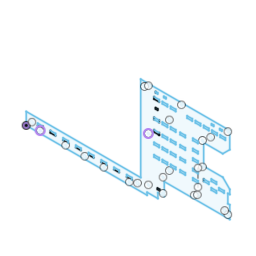
R&S UPL KeyBoard BackPanel (Autodesk Fusion 360 design; units mm, degrees)
description: Rohde & Schwarz UPL
Autodesk Fusion 360 part; units mm, degrees
sketch "Mechanical Outline" plane through (0, 0, 0) normal (0, 0, 1) x (1, 0, 0)
  line L0 (180, 19) -> (0, 19)
  line L1 (309, 116) -> (279, 116)
  line L2 (279, 116) -> (279, 84)
  line L3 (279, 84) -> (309, 84)
  line L4 (309, 84) -> (320, 73)
  line L5 (320, 66) -> (317, 66)
  line L6 (317, 66) -> (317, 52)
  line L7 (317, 52) -> (320, 52)
  line L8 (320, 66) -> (320, 73)
  line L9 (320, 32) -> (217, 32)
  line L10 (190, 0) -> (0, 0)
  line L11 (0, 19) -> (0, 0)
  line L12 (320, 52) -> (320, 32)
  line L13 (207, 4) -> (190, 4)
  line L14 (190, 4) -> (190, 0)
  line L15 (207, 12) -> (217, 12)
  line L16 (207, 12) -> (207, 4)
  line L17 (217, 32) -> (217, 12)
  line L18 (320, 153) -> (180, 153)
  line L19 (180, 19) -> (180, 153)
  line L20 (320, 153) -> (320, 127)
  line L21 (309, 116) -> (320, 127)
  dimension "d21" = 3
  dimension "d22" = 14
  dimension "d124" = 19
  dimension "d126" = 103
  dimension "d130" = 4
  dimension "d131" = 8
  dimension "d132" = 20
  dimension "d133" = 17
  dimension "d134" = 10
  constraint horizontal L1
  constraint vertical L2
  constraint horizontal L3
  constraint horizontal L5
  constraint vertical L6
  constraint horizontal L7
  constraint horizontal L9
  constraint horizontal L10
  constraint perpendicular L10 L11
  constraint horizontal L13
  constraint perpendicular L10 L14
  constraint horizontal L15
  constraint horizontal L18
  constraint perpendicular L18 L19
  measures "d21" distance of L5.start L5.end
  measures "d22" distance of L5.start L7.end
  measures "d124" distance of L0.end L10.end
  measures "d126" distance of L9.start L9.end
  measures "d130" distance of L10.start L13.end
  measures "d131" distance of L13.start L15.start
  measures "d132" distance of L9.end L15.end
  measures "d133" distance of L13.start L13.end
  measures "d134" distance of L15.start L15.end
sketch "Holes" plane through (0, 0, 0) normal (0, 0, 1) x (1, 0, 0)
  circle A0 centre (175, 9) radius 2
  circle A1 centre (186, 146) radius 2
  circle A2 centre (92, 4) radius 2
  circle A3 centre (9, 9) radius 2
  circle A4 centre (22, 4) radius 1.25
  circle A5 centre (62, 4) radius 1.25
  circle A6 centre (122, 4) radius 1.25
  circle A7 centre (162, 4) radius 1.25
  circle A8 centre (192, 150) radius 1.25
  circle A9 centre (192, 85) radius 1.25
  circle A10 centre (192, 15) radius 1.25
  circle A11 centre (244, 150) radius 1.25
  circle A12 centre (317, 150) radius 1.25
  circle A13 centre (225, 120) radius 2
  circle A14 centre (290, 129) radius 2
  circle A15 centre (225, 51) radius 2
  circle A16 centre (277, 118) radius 1.25
  circle A17 centre (277, 82) radius 1.25
  circle A18 centre (215, 15) radius 1.25
  circle A19 centre (215, 37) radius 1.25
  circle A20 centre (264, 37) radius 1.25
  circle A21 centre (317, 37) radius 1.25
  circle A22 centre (269, 40) radius 2
  circle A23 centre (312, 40) radius 2
  dimension "d28" = 4
  dimension "d31" = 4
  dimension "d39" = 4
  dimension "d40" = 4
  dimension "d41" = 2.5
  dimension "d43" = 2.5
  dimension "d44" = 2.5
  dimension "d51" = 13
  dimension "d52" = 40
  dimension "d53" = 30
  dimension "d55" = 40
  dimension "d56" = 13
  dimension "d60" = 2.5
  dimension "d61" = 6
  dimension "d62" = 4
  dimension "d63" = 2.5
  dimension "d66" = 2.5
  dimension "d69" = 2.5
  dimension "d70" = 2.5
  dimension "d73" = 52
  dimension "d75" = 4
  dimension "d76" = 4
  dimension "d77" = 4
  dimension "d78" = 39
  dimension "d79" = 104
  dimension "d80" = 17
  dimension "d81" = 26
  dimension "d82" = 95
  dimension "d84" = 2.5
  dimension "d85" = 2.5
  dimension "d86" = 91
  dimension "d88" = 28
  dimension "d89" = 64
  dimension "d90" = 2.5
  dimension "d91" = 2.5
  dimension "d92" = 2.5
  dimension "d93" = 2.5
  dimension "d94" = 4
  dimension "d95" = 4
  dimension "d111" = 60
  dimension "d112" = 65
  dimension "d113" = 70
  dimension "d114" = 73
  dimension "d115" = 22
  dimension "d116" = 49
  dimension "d117" = 53
  dimension "d118" = 23
  dimension "d119" = 44
  dimension "d120" = 43
  dimension "d121" = 11
  dimension "d122" = 2.5
  constraint horizontal A10.centre A18.centre
  constraint vertical A18.centre A19.centre
  constraint horizontal A19.centre A20.centre
  constraint horizontal A20.centre A21.centre
  constraint vertical A16.centre A17.centre
  constraint horizontal A6.centre A7.centre
  constraint horizontal A4.centre A5.centre
  constraint horizontal A0.centre A3.centre
  constraint horizontal A8.centre A11.centre
  constraint horizontal A11.centre A12.centre
  constraint vertical A13.centre A15.centre
  constraint vertical A8.centre A9.centre
  constraint horizontal A22.centre A23.centre
  measures "d28" diameter of A0
  measures "d31" diameter of A1
  measures "d39" diameter of A2
  measures "d40" diameter of A3
  measures "d41" diameter of A4
  measures "d43" diameter of A6
  measures "d44" diameter of A7
  measures "d51" horizontal distance of A0.centre A7.centre
  measures "d52" distance of A6.centre A7.centre
  measures "d53" horizontal distance of A2.centre A6.centre
  measures "d55" distance of A4.centre A5.centre
  measures "d56" horizontal distance of A3.centre A4.centre
  measures "d60" diameter of A8
  measures "d61" horizontal distance of A1.centre A8.centre
  measures "d62" vertical distance of A1.centre A8.centre
  measures "d63" diameter of A9
  measures "d66" diameter of A10
  measures "d69" diameter of A11
  measures "d70" diameter of A12
  measures "d73" distance of A8.centre A11.centre
  measures "d75" diameter of A13
  measures "d76" diameter of A14
  measures "d77" diameter of A15
  measures "d78" horizontal distance of A1.centre A13.centre
  measures "d79" horizontal distance of A1.centre A14.centre
  measures "d80" vertical distance of A1.centre A14.centre
  measures "d81" vertical distance of A1.centre A13.centre
  measures "d82" vertical distance of A1.centre A15.centre
  measures "d84" diameter of A16
  measures "d85" diameter of A17
  measures "d86" horizontal distance of A1.centre A16.centre
  measures "d88" vertical distance of A1.centre A16.centre
  measures "d89" vertical distance of A1.centre A17.centre
  measures "d90" diameter of A18
  measures "d91" diameter of A19
  measures "d92" diameter of A20
  measures "d93" diameter of A21
  measures "d94" diameter of A22
  measures "d95" diameter of A23
  measures "d111" distance of A5.centre A6.centre
  measures "d112" distance of A8.centre A9.centre
  measures "d113" distance of A9.centre A10.centre
  measures "d114" distance of A11.centre A12.centre
  measures "d115" distance of A18.centre A19.centre
  measures "d116" distance of A19.centre A20.centre
  measures "d117" distance of A20.centre A21.centre
  measures "d118" distance of A10.centre A18.centre
  measures "d119" horizontal distance of A15.centre A22.centre
  measures "d120" distance of A22.centre A23.centre
  measures "d121" vertical distance of A15.centre A22.centre
  measures "d122" diameter of A5
extrude "Extrude1" add sketch "Mechanical Outline" along normal blind 1
sketch "Buttons/Leds" plane through (0, 0, 0) normal (0, 0, 1) x (1, 0, 0)
  line L0 (26, 12) -> (26, 9)
  line L1 (58, 9) -> (66, 9)
  line L2 (106, 12) -> (106, 9)
  line L3 (86, 12) -> (86, 9)
  line L4 (66, 12) -> (58, 12)
  line L5 (46, 9) -> (38, 9)
  line L6 (26, 9) -> (18, 9)
  line L7 (86, 9) -> (78, 9)
  line L8 (66, 9) -> (66, 12)
  line L9 (18, 9) -> (18, 12)
  line L10 (106, 9) -> (98, 9)
  line L11 (138, 12) -> (146, 12)
  line L12 (146, 12) -> (146, 9)
  line L13 (118, 12) -> (126, 12)
  line L14 (138, 9) -> (138, 12)
  line L15 (158, 9) -> (158, 12)
  line L16 (166, 12) -> (166, 9)
  line L17 (98, 12) -> (106, 12)
  line L18 (126, 12) -> (126, 9)
  line L19 (158, 12) -> (166, 12)
  line L20 (146, 9) -> (138, 9)
  line L21 (166, 9) -> (158, 9)
  line L22 (18, 12) -> (26, 12)
  line L23 (78, 9) -> (78, 12)
  line L24 (78, 12) -> (86, 12)
  line L25 (58, 12) -> (58, 9)
  line L26 (38, 9) -> (38, 12)
  line L27 (46, 12) -> (46, 9)
  line L28 (38, 12) -> (46, 12)
  line L29 (98, 9) -> (98, 12)
  line L30 (126, 9) -> (118, 9)
  line L31 (118, 9) -> (118, 12)
  line L32 (214, 111.5) -> (222, 111.5)
  line L33 (227, 77.5) -> (235, 77.5)
  line L34 (242, 108.5) -> (242, 111.5)
  line L35 (235, 108.5) -> (227, 108.5)
  line L36 (235, 74.5) -> (227, 74.5)
  line L37 (250, 94.5) -> (250, 91.5)
  line L38 (235, 91.5) -> (227, 91.5)
  line L39 (222, 60.5) -> (222, 57.5)
  line L40 (270, 110.5) -> (262, 110.5)
  line L41 (270, 96.5) -> (262, 96.5)
  line L42 (262, 83.5) -> (262, 86.5)
  line L43 (262, 113.5) -> (270, 113.5)
  line L44 (262, 96.5) -> (262, 99.5)
  line L45 (262, 110.5) -> (262, 113.5)
  line L46 (270, 59.5) -> (270, 56.5)
  line L47 (270, 99.5) -> (270, 96.5)
  line L48 (262, 69.5) -> (262, 72.5)
  line L49 (270, 72.5) -> (270, 69.5)
  line L50 (262, 59.5) -> (270, 59.5)
  line L51 (262, 86.5) -> (270, 86.5)
  line L52 (270, 69.5) -> (262, 69.5)
  line L53 (270, 86.5) -> (270, 83.5)
  line L54 (262, 72.5) -> (270, 72.5)
  line L55 (270, 56.5) -> (262, 56.5)
  line L56 (270, 83.5) -> (262, 83.5)
  line L57 (262, 56.5) -> (262, 59.5)
  line L58 (270, 113.5) -> (270, 110.5)
  line L59 (262, 99.5) -> (270, 99.5)
  line L60 (250, 57.5) -> (242, 57.5)
  line L61 (242, 111.5) -> (250, 111.5)
  line L62 (209, 77.5) -> (209, 74.5)
  line L63 (242, 60.5) -> (250, 60.5)
  line L64 (227, 111.5) -> (235, 111.5)
  line L65 (201, 94.5) -> (209, 94.5)
  line L66 (227, 60.5) -> (235, 60.5)
  line L67 (201, 77.5) -> (209, 77.5)
  line L68 (235, 57.5) -> (227, 57.5)
  line L69 (214, 74.5) -> (214, 77.5)
  line L70 (222, 108.5) -> (214, 108.5)
  line L71 (222, 111.5) -> (222, 108.5)
  line L72 (214, 60.5) -> (222, 60.5)
  line L73 (222, 91.5) -> (214, 91.5)
  line L74 (250, 111.5) -> (250, 108.5)
  line L75 (227, 108.5) -> (227, 111.5)
  line L76 (222, 94.5) -> (222, 91.5)
  line L77 (222, 57.5) -> (214, 57.5)
  line L78 (250, 74.5) -> (242, 74.5)
  line L79 (209, 60.5) -> (209, 57.5)
  line L80 (227, 57.5) -> (227, 60.5)
  line L81 (209, 91.5) -> (201, 91.5)
  line L82 (235, 60.5) -> (235, 57.5)
  line L83 (235, 94.5) -> (235, 91.5)
  line L84 (214, 57.5) -> (214, 60.5)
  line L85 (201, 57.5) -> (201, 60.5)
  line L86 (201, 60.5) -> (209, 60.5)
  line L87 (250, 91.5) -> (242, 91.5)
  line L88 (209, 57.5) -> (201, 57.5)
  line L89 (201, 111.5) -> (209, 111.5)
  line L90 (209, 111.5) -> (209, 108.5)
  line L91 (201, 74.5) -> (201, 77.5)
  line L92 (214, 108.5) -> (214, 111.5)
  line L93 (242, 91.5) -> (242, 94.5)
  line L94 (242, 57.5) -> (242, 60.5)
  line L95 (250, 108.5) -> (242, 108.5)
  line L96 (214, 91.5) -> (214, 94.5)
  line L97 (235, 111.5) -> (235, 108.5)
  line L98 (250, 60.5) -> (250, 57.5)
  line L99 (214, 77.5) -> (222, 77.5)
  line L100 (209, 94.5) -> (209, 91.5)
  line L101 (209, 108.5) -> (201, 108.5)
  line L102 (209, 74.5) -> (201, 74.5)
  line L103 (201, 108.5) -> (201, 111.5)
  line L104 (222, 74.5) -> (214, 74.5)
  line L105 (227, 74.5) -> (227, 77.5)
  line L106 (227, 91.5) -> (227, 94.5)
  line L107 (222, 77.5) -> (222, 74.5)
  line L108 (235, 77.5) -> (235, 74.5)
  line L109 (242, 94.5) -> (250, 94.5)
  line L110 (250, 77.5) -> (250, 74.5)
  line L111 (242, 77.5) -> (250, 77.5)
  line L112 (214, 94.5) -> (222, 94.5)
  line L113 (227, 94.5) -> (235, 94.5)
  line L114 (242, 74.5) -> (242, 77.5)
  line L115 (201, 94.5) -> (201, 91.5)
  line L116 (209, 91.5) -> (208.5, 91.5)
  line L117 (291, 69.5) -> (291, 72.5)
  line L118 (311, 63.5) -> (303, 63.5)
  line L119 (270, 77) -> (270, 51) construction
  line L120 (279, 66.5) -> (287, 66.5)
  line L121 (287, 66.5) -> (287, 63.5)
  line L122 (287, 63.5) -> (279, 63.5)
  line L123 (279, 63.5) -> (279, 66.5)
  line L124 (291, 72.5) -> (299, 72.5)
  line L125 (299, 72.5) -> (299, 69.5)
  line L126 (291, 60.5) -> (299, 60.5)
  line L127 (299, 60.5) -> (299, 57.5)
  line L128 (299, 57.5) -> (291, 57.5)
  line L129 (303, 66.5) -> (311, 66.5)
  line L130 (311, 66.5) -> (311, 63.5)
  line L131 (291, 57.5) -> (291, 60.5)
  line L132 (291, 69.5) -> (299, 69.5)
  line L133 (303, 66.5) -> (303, 63.5)
  line L134 (235, 139.5) -> (235, 136.5)
  line L135 (227, 139.5) -> (235, 139.5)
  line L136 (235, 136.5) -> (227, 136.5)
  line L137 (274, 139.5) -> (274, 136.5)
  line L138 (222, 136.5) -> (222, 139.5)
  line L139 (227, 136.5) -> (227, 139.5)
  line L140 (201, 136.5) -> (201, 139.5)
  line L141 (203.4, 146.2) -> (203.4, 147.8)
  line L142 (214, 139.5) -> (214, 136.5)
  line L143 (266, 136.5) -> (266, 139.5)
  line L144 (304.4, 146.2) -> (304.4, 147.8)
  line L145 (294.6, 147.8) -> (294.6, 146.2)
  line L146 (253, 136.5) -> (253, 139.5)
  line L147 (287, 139.5) -> (287, 136.5)
  line L148 (206.6, 147.8) -> (206.6, 146.2)
  line L149 (266, 139.5) -> (274, 139.5)
  line L150 (279, 139.5) -> (287, 139.5)
  line L151 (209, 136.5) -> (201, 136.5)
  line L152 (216.4, 146.2) -> (216.4, 147.8)
  line L153 (219.6, 147.8) -> (219.6, 146.2)
  line L154 (216.4, 147.8) -> (219.6, 147.8)
  line L155 (307.6, 146.2) -> (304.4, 146.2)
  line L156 (201, 139.5) -> (209, 139.5)
  line L157 (305, 139.5) -> (313, 139.5)
  line L158 (219.6, 146.2) -> (216.4, 146.2)
  line L159 (203.4, 147.8) -> (206.6, 147.8)
  line L160 (206.6, 146.2) -> (203.4, 146.2)
  line L161 (209, 139.5) -> (209, 136.5)
  line L162 (287, 136.5) -> (279, 136.5)
  line L163 (291.4, 147.8) -> (294.6, 147.8)
  line L164 (292, 136.5) -> (292, 139.5)
  line L165 (274, 136.5) -> (266, 136.5)
  line L166 (253, 139.5) -> (261, 139.5)
  line L167 (300, 136.5) -> (292, 136.5)
  line L168 (294.6, 146.2) -> (291.4, 146.2)
  line L169 (291.4, 146.2) -> (291.4, 147.8)
  line L170 (261, 136.5) -> (253, 136.5)
  line L171 (279, 136.5) -> (279, 139.5)
  line L172 (313, 139.5) -> (313, 136.5)
  line L173 (307.6, 147.8) -> (307.6, 146.2)
  line L174 (222, 139.5) -> (214, 139.5)
  line L175 (313, 136.5) -> (305, 136.5)
  line L176 (214, 136.5) -> (222, 136.5)
  line L177 (261, 139.5) -> (261, 136.5)
  line L178 (305, 136.5) -> (305, 139.5)
  line L179 (292, 139.5) -> (300, 139.5)
  line L180 (300, 139.5) -> (300, 136.5)
  line L181 (304.4, 147.8) -> (307.6, 147.8)
  line L182 (206.6, 125.8) -> (203.4, 125.8)
  line L183 (203.4, 125.8) -> (203.4, 124.2)
  line L184 (203.4, 124.2) -> (206.6, 124.2)
  line L185 (206.6, 124.2) -> (206.6, 125.8)
  line L186 (209.6, 16.2) -> (209.6, 17.8)
  line L187 (206.4, 17.8) -> (206.4, 16.2)
  line L188 (209.6, 17.8) -> (206.4, 17.8)
  line L189 (206.4, 16.2) -> (209.6, 16.2)
  point P0 (22, 4)
  point P1 (192, 85)
  dimension "d142" = 4
  dimension "d143" = 5
  dimension "d144" = 5
  dimension "d145" = 12
  dimension "d147" = 12
  dimension "d148" = 5
  dimension "d149" = 12
  dimension "d150" = 5
  dimension "d151" = 12
  dimension "d153" = 5
  dimension "d154" = 12
  dimension "d155" = 5
  dimension "d156" = 12
  dimension "d157" = 5
  dimension "d158" = 12
  dimension "d159" = 5
  dimension "d160" = 5
  dimension "d161" = 5
  dimension "d162" = 5
  dimension "d163" = 5
  dimension "d164" = 5
  dimension "d165" = 5
  dimension "d166" = 5
  dimension "d167" = 5
  dimension "d168" = 7
  dimension "d169" = 7
  dimension "d170" = 7
  dimension "d171" = 7
  dimension "d172" = 12
  dimension "d173" = 12
  dimension "d174" = 12
  dimension "d175" = 12
  dimension "d176" = 12
  dimension "d177" = 14
  dimension "d178" = 14
  dimension "d179" = 14
  dimension "d180" = 14
  dimension "d181" = 14
  dimension "d182" = 14
  dimension "d183" = 14
  dimension "d184" = 14
  dimension "d185" = 14
  dimension "d186" = 14
  dimension "d187" = 14
  dimension "d188" = 14
  dimension "d189" = 11
  dimension "d190" = 10
  dimension "d191" = 11
  dimension "d192" = 10
  dimension "d193" = 2
  dimension "d194" = 5
  dimension "d195" = 9
  dimension "d196" = 12
  dimension "d197" = 1
  dimension "d198" = 6.5
  dimension "d199" = 9
  dimension "d244" = 8
  dimension "d245" = 3
  dimension "d248" = 8
  dimension "d249" = 8
  dimension "d250" = 8
  dimension "d251" = 8
  dimension "d252" = 8
  dimension "d253" = 8
  dimension "d254" = 8
  dimension "d255" = 8
  dimension "d256" = 8
  dimension "d257" = 8
  dimension "d258" = 8
  dimension "d259" = 8
  dimension "d260" = 8
  dimension "d261" = 8
  dimension "d262" = 8
  dimension "d263" = 8
  dimension "d264" = 8
  dimension "d265" = 8
  dimension "d266" = 8
  dimension "d267" = 8
  dimension "d268" = 3
  dimension "d269" = 3
  dimension "d270" = 3
  dimension "d271" = 3
  dimension "d274" = 3
  dimension "d275" = 3
  dimension "d276" = 9
  dimension "d278" = 12
  dimension "d279" = 78
  dimension "d281" = 9
  dimension "d282" = 4
  dimension "d283" = 4
  dimension "d284" = 4
  dimension "d285" = 4
  dimension "d286" = 3
  dimension "d287" = 3
  dimension "d288" = 3
  dimension "d289" = 3
  dimension "d290" = 3
  dimension "d291" = 6.7
  dimension "d292" = 6.7
  dimension "d293" = 6.7
  dimension "d294" = 6.7
  dimension "d295" = 2.4
  dimension "d296" = 5
  dimension "d297" = 5
  dimension "d298" = 9.8
  dimension "d299" = 18
  dimension "d300" = 5
  dimension "d301" = 5
  dimension "d302" = 5
  dimension "d303" = 5
  dimension "d305" = 9
  dimension "d306" = 51.5
  dimension "d307" = 3.2
  dimension "d308" = 1.6
  dimension "d309" = 10.7
  dimension "d311" = 2.4
  dimension "d312" = 3.2
  dimension "d313" = 1.6
  dimension "d314" = 67.2
  dimension "d315" = 14.4
  dimension "d317" = 71.8
  dimension "d318" = 9.8
  constraint horizontal L6
  constraint horizontal L5
  constraint horizontal L1
  constraint horizontal L7
  constraint horizontal L10
  constraint vertical L26
  constraint vertical L0
  constraint vertical L9
  constraint vertical L27
  constraint vertical L25
  constraint vertical L8
  constraint vertical L23
  constraint vertical L3
  constraint vertical L29
  constraint horizontal L22
  constraint horizontal L28
  constraint horizontal L4
  constraint horizontal L24
  constraint horizontal L17
  constraint vertical L2
  constraint vertical L31
  constraint horizontal L13
  constraint vertical L18
  constraint horizontal L30
  constraint horizontal L11
  constraint horizontal L20
  constraint vertical L14
  constraint vertical L12
  constraint vertical L15
  constraint horizontal L19
  constraint horizontal L21
  constraint vertical L16
  constraint vertical L103
  constraint horizontal L101
  constraint horizontal L89
  constraint vertical L90
  constraint horizontal L65
  constraint vertical L100
  constraint horizontal L81
  constraint horizontal L67
  constraint horizontal L102
  constraint vertical L91
  constraint vertical L62
  constraint horizontal L86
  constraint horizontal L88
  constraint vertical L85
  constraint vertical L79
  constraint vertical L84
  constraint horizontal L77
  constraint horizontal L72
  constraint vertical L39
  constraint horizontal L104
  constraint horizontal L99
  constraint vertical L107
  constraint vertical L69
  constraint horizontal L73
  constraint horizontal L112
  constraint vertical L96
  constraint vertical L76
  constraint horizontal L70
  constraint horizontal L32
  constraint vertical L92
  constraint vertical L71
  constraint vertical L75
  constraint horizontal L64
  constraint horizontal L35
  constraint vertical L97
  constraint horizontal L113
  constraint vertical L106
  constraint horizontal L38
  constraint vertical L83
  constraint horizontal L33
  constraint horizontal L36
  constraint vertical L105
  constraint vertical L108
  constraint horizontal L66
  constraint horizontal L68
  constraint vertical L80
  constraint vertical L82
  constraint vertical L94
  constraint horizontal L63
  constraint horizontal L60
  constraint vertical L98
  constraint horizontal L78
  constraint horizontal L111
  constraint vertical L110
  constraint vertical L114
  constraint horizontal L87
  constraint horizontal L109
  constraint vertical L37
  constraint vertical L93
  constraint horizontal L95
  constraint horizontal L61
  constraint vertical L74
  constraint vertical L34
  constraint vertical L45
  constraint horizontal L43
  constraint horizontal L40
  constraint vertical L58
  constraint horizontal L59
  constraint horizontal L41
  constraint vertical L44
  constraint vertical L47
  constraint horizontal L51
  constraint horizontal L56
  constraint vertical L42
  constraint vertical L53
  constraint horizontal L54
  constraint horizontal L52
  constraint vertical L48
  constraint vertical L49
  constraint horizontal L50
  constraint horizontal L55
  constraint vertical L46
  constraint vertical L57
  constraint perpendicular L81 L115
  constraint coincident L81 L116.end
  constraint vertical L117
  constraint horizontal L118
  constraint vertical L119
  constraint horizontal L120
  constraint vertical L121
  constraint horizontal L122
  constraint vertical L123
  constraint horizontal L124
  constraint vertical L125
  constraint horizontal L126
  constraint vertical L127
  constraint horizontal L128
  constraint horizontal L129
  constraint vertical L130
  constraint perpendicular L126 L131
  constraint perpendicular L125 L132
  constraint perpendicular L118 L133
  constraint vertical L140
  constraint horizontal L156
  constraint horizontal L151
  constraint vertical L161
  constraint horizontal L160
  constraint horizontal L159
  constraint vertical L148
  constraint vertical L141
  constraint vertical L152
  constraint horizontal L154
  constraint horizontal L158
  constraint vertical L153
  constraint horizontal L174
  constraint horizontal L176
  constraint vertical L142
  constraint vertical L138
  constraint vertical L139
  constraint horizontal L135
  constraint horizontal L136
  constraint vertical L134
  constraint vertical L146
  constraint horizontal L170
  constraint vertical L177
  constraint horizontal L166
  constraint horizontal L149
  constraint horizontal L165
  constraint vertical L143
  constraint vertical L137
  constraint vertical L171
  constraint horizontal L150
  constraint horizontal L162
  constraint vertical L147
  constraint horizontal L168
  constraint horizontal L163
  constraint vertical L169
  constraint vertical L145
  constraint horizontal L179
  constraint horizontal L167
  constraint vertical L164
  constraint vertical L180
  constraint vertical L178
  constraint horizontal L157
  constraint horizontal L175
  constraint vertical L172
  constraint horizontal L155
  constraint horizontal L181
  constraint vertical L173
  constraint vertical L144
  constraint horizontal L182
  constraint horizontal L184
  constraint vertical L185
  constraint vertical L183
  constraint vertical L187
  constraint horizontal L188
  constraint horizontal L189
  constraint vertical L186
  measures "d142" horizontal distance of L0.end P0
  measures "d143" vertical distance of L6.end P0
  measures "d144" distance of L5 P0
  measures "d145" distance of L26.end L0
  measures "d147" horizontal distance of L4.end L27.start
  measures "d148" distance of L1 P0
  measures "d149" horizontal distance of L4.start L23.end
  measures "d150" vertical distance of L7.end P0
  measures "d151" horizontal distance of L17.start L3.start
  measures "d153" vertical distance of L10.end P0
  measures "d154" horizontal distance of L13.start L2.start
  measures "d155" vertical distance of L30.end P0
  measures "d156" horizontal distance of L11.start L13.end
  measures "d157" vertical distance of L14.start P0
  measures "d158" horizontal distance of L11.end L15.end
  measures "d159" distance of L21 P0
  measures "d160" distance of L32.start L89.end
  measures "d161" distance of L65.end L96.end
  measures "d162" distance of L69.end L62.start
  measures "d163" distance of L72.start L79.start
  measures "d164" distance of L39.start L66.start
  measures "d165" distance of L99.end L33.start
  measures "d166" distance of L106.end L76.start
  measures "d167" distance of L64.start L32.end
  measures "d168" distance of L34.end L64.end
  measures "d169" distance of L83.start L93.end
  measures "d170" distance of L33.end L111.start
  measures "d171" distance of L66.end L63.start
  measures "d172" horizontal distance of L50.start L63.end
  measures "d173" horizontal distance of L110.start L48.end
  measures "d174" horizontal distance of L42.start L37.end
  measures "d175" distance of L74.end L44
  measures "d176" horizontal distance of L74.end L40.end
  measures "d177" distance of L101.end L65.start
  measures "d178" distance of L67.start L81.end
  measures "d179" distance of L91.start L85.end
  measures "d180" distance of L70.end L112
  measures "d181" distance of L73.end L69.end
  measures "d182" distance of L72.start L69.start
  measures "d183" distance of L106.end L35.end
  measures "d184" distance of L38.end L33.start
  measures "d185" distance of L36.end L66.start
  measures "d186" distance of L78.end L63.start
  measures "d187" distance of L87.end L111.start
  measures "d188" distance of L34.start L93.end
  measures "d189" distance of L40.end L44.end
  measures "d190" distance of L42.end L41.end
  measures "d191" distance of L42.start L48.end
  measures "d192" distance of L50.start L48.start
  measures "d193" vertical distance of L61.end L43.start
  measures "d194" vertical distance of L44.end L37.start
  measures "d195" vertical distance of L110.start L42.end
  measures "d196" vertical distance of L48.end L63.end
  measures "d197" vertical distance of L55.end L60.start
  measures "d198" vertical distance of L81.end P1
  measures "d199" horizontal distance of L81.end P1
  measures "d244" distance of L49.start L48.end
  measures "d245" distance of L49.start L49.end
  measures "d248" distance of L79.end L85.start
  measures "d249" distance of L39.end L77.end
  measures "d250" distance of L68.start L68.end
  measures "d251" distance of L60.end L60.start
  measures "d252" distance of L55.end L46.end
  measures "d253" distance of L78.end L78.start
  measures "d254" distance of L36.end L36.start
  measures "d255" distance of L104.start L69.start
  measures "d256" distance of L91.start L62.end
  measures "d257" distance of L81.start L81.end
  measures "d258" distance of L73.start L73.end
  measures "d259" distance of L38.end L38.start
  measures "d260" distance of L87.end L37.end
  measures "d261" distance of L42.end L51.end
  measures "d262" distance of L44.end L47.start
  measures "d263" distance of L34.start L74.end
  measures "d264" distance of L40.start L40.end
  measures "d265" distance of L35.end L35.start
  measures "d266" distance of L70.start L70.end
  measures "d267" distance of L90.end L101.end
  measures "d268" distance of L101.end L89.start
  measures "d269" distance of L32.start L70.end
  measures "d270" distance of L64.start L35.end
  measures "d271" distance of L34.end L34.start
  measures "d274" distance of L67.start L91.start
  measures "d275" distance of L85.start L85.end
  measures "d276" distance of L103 P1
  measures "d278" distance of L42 L110
  measures "d279" distance of P1 L119
  measures "d281" distance of L119 L123
  measures "d282" distance of L117 L121
  measures "d283" distance of L125 L133
  measures "d284" distance of L121 L131
  measures "d285" distance of L127 L133
  measures "d286" distance of L120 L132
  measures "d287" distance of L122 L126
  measures "d288" distance of L118 L126
  measures "d289" distance of L129 L132
  measures "d290" distance of L52 L120
  measures "d291" distance of L156 L160
  measures "d292" distance of L158 L174
  measures "d293" distance of L168 L179
  measures "d294" distance of L155 L157
  measures "d295" distance of L140 L141
  measures "d296" distance of L142 L161
  measures "d297" distance of L138 L139
  measures "d298" distance of L148 L152
  measures "d299" distance of L134 L146
  measures "d300" distance of L143 L177
  measures "d301" distance of L137 L171
  measures "d302" distance of L147 L164
  measures "d303" distance of L178 L180
  measures "d305" distance of P1 L140
  measures "d306" distance of P1 L151
  measures "d307" distance of L182.start L182.end
  measures "d308" distance of L184.end L182.start
  measures "d309" distance of L151 L182.start
  measures "d311" distance of L140 L182.end
  measures "d312" distance of L186.end L187.start
  measures "d313" distance of L186.start L186.end
  measures "d314" vertical distance of P1 L187.start
  measures "d315" horizontal distance of P1 L187.start
  measures "d317" distance of L163.start L153.start
  measures "d318" distance of L144 L145
hidden bodies 1
equation "d28 = d40"
equation "d31 = d40"
equation "d39 = d40"
equation "d43 = d41"
equation "d44 = d41"
equation "d60 = d41"
equation "d63 = d41"
equation "d66 = d41"
equation "d69 = d41"
equation "d70 = d41"
equation "d75 = d40"
equation "d76 = d40"
equation "d77 = d40"
equation "d84 = d41"
equation "d85 = d41"
equation "d90 = d41"
equation "d91 = d41"
equation "d92 = d41"
equation "d93 = d41"
equation "d94 = d40"
equation "d95 = d40"
equation "d122 = d41"
